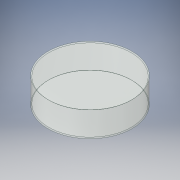
# Autodesk Inventor part: Tank
Saved by Autodesk Inventor 2017 (Build 210142000, 142)
## iProperties
Part Number: Tank
Material: Glas
Document SubType Name: Modeling
Designer: OleSi
Density: 2.18 g/cm^3
Appearance: Klar
Mass: 392.699 g
Surface Area: 314.159 cm^2
Volume: 392.699 cm^3
Author: OleSi
Autodesk Inventor part; units mm, degrees
ref_plane "YZ Plane" through (0, 0, 0) normal (1, 0, 0) x (0, 1, 0)
ref_plane "XZ Plane" through (0, 0, 0) normal (0, 1, 0) x (-1, 0, 0)
ref_plane "XY Plane" through (0, 0, 0) normal (0, 0, 1) x (1, 0, 0)
sketch "Skizze2" plane through (0, 0, 0) normal (0, 0, 1) x (1, 0, 0)
  circle A0 centre (0, 0) radius 50
  dimension "d2" = 100
  constraints: 1 centre point, 1 coincident
  measures "d2" diameter of A0
extrude "Extrusion1" add sketch "Skizze2" along normal blind 30
shell "Wandung1" thickness 1 removed faces 0
